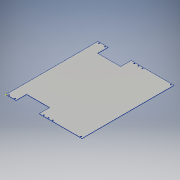
# Autodesk Inventor part: Belly Pan
Saved by Autodesk Inventor 2018 (Build 220112000, 112)
## iProperties
Created: 2018-01-27
Part Number: Belly Pan
Material: Aluminum 6061
Document SubType Name: Modeling
Designer: s-4000369
Density: 2.7 g/cm^3
Appearance: Aluminum - Flat
Mass: 1648.73 g
Surface Area: 4866.5 cm^2
Volume: 610.641 cm^3
Author: s-4000369
Autodesk Inventor part; units mm, degrees
ref_plane "YZ Plane" through (0, 0, 0) normal (1, 0, 0) x (0, 1, 0)
ref_plane "XZ Plane" through (0, 0, 0) normal (0, 1, 0) x (-1, 0, 0)
ref_plane "XY Plane" through (0, 0, 0) normal (0, 0, 1) x (1, 0, 0)
sketch "Sketch1" plane through (0, 0, 0) normal (0, 1, 0) x (-1, 0, 0)
  point P0 (0, 0)
sketch "Sketch2" plane through (0, 0, 0) normal (0, 1, 0) x (-1, 0, 0)
  line L0 (-61.9252, 0) -> (0, 0)
  line L1 (0, 0) -> (0, -558.8)
  line L2 (0, -558.8) -> (-61.9252, -558.8)
  line L3 (-61.9252, -558.8) -> (-61.9252, -495.3)
  line L4 (-61.9252, -495.3) -> (-201.6252, -495.3)
  line L5 (-201.6252, -495.3) -> (-201.6252, -558.8)
  line L6 (-201.6252, -558.8) -> (-461.9752, -558.8)
  line L7 (-461.9752, -558.8) -> (-461.9752, 0)
  line L8 (-461.9752, 0) -> (-201.6252, 0)
  line L9 (-201.6252, 0) -> (-201.6252, -63.5)
  line L10 (-201.6252, -63.5) -> (-61.9252, -63.5)
  line L11 (-61.9252, -63.5) -> (-61.9252, 0)
  point P0 (0, 0)
  dimension "d1" = 558.8
  dimension "d2" = 139.7
  dimension "d3" = 61.9252
  dimension "d4" = 63.5
  dimension "d8" = 260.35
  constraints: 24 end point, 8 perpendicular, 5 point on line, 2 collinear, 1 coincident, 1 horizontal, 1 vertical
  measures "d1" distance between parallel lines of L6 L8
  measures "d2" distance of L9.end L10.end
  measures "d3" distance of L0.start L0.end
  measures "d4" distance of L8.end L9.end
  measures "d8" distance of L7.end L8.end
extrude "Extrusion1" add sketch "Sketch2" along normal blind 1.5875
sketch "Sketch3" plane through (0, 1.5875, 0) normal (0, 1, 0) x (1, 0, 0)
  line L0 (461.9752, 0) -> (461.9752, 558.8) projected
  line L1 (461.9752, 0) -> (461.9752, 12.7)
  line L2 (461.9752, 12.7) -> (201.6252, 12.7)
  line L3 (201.6252, 63.5) -> (201.6252, 0) projected
  line L4 (201.6252, 558.8) -> (461.9752, 558.8) projected
  line L5 (461.9752, 558.8) -> (461.9752, 546.1)
  line L6 (461.9752, 546.1) -> (201.6252, 546.1)
  line L7 (201.6252, 558.8) -> (201.6252, 495.3) projected
  line L8 (461.9752, 6.35) -> (201.6252, 6.35)
  line L9 (461.9752, 552.45) -> (201.6252, 552.45)
  line L10 (461.9752, 552.45) -> (449.2752, 552.45)
  line L11 (461.9752, 6.35) -> (449.2752, 6.35)
  line L12 (201.6252, 552.45) -> (227.0252, 552.45)
  line L13 (227.0252, 552.45) -> (252.4252, 552.45)
  line L14 (252.4252, 552.45) -> (277.8252, 552.45)
  line L15 (201.6252, 6.35) -> (227.0252, 6.35)
  line L16 (227.0252, 6.35) -> (252.4252, 6.35)
  line L17 (252.4252, 6.35) -> (277.8252, 6.35)
  line L18 (0, 558.8) -> (0, 0) projected
  line L19 (0, 552.45) -> (62.0515, 552.45)
  line L20 (0, 6.35) -> (62.0515, 6.35)
  line L21 (0, 552.45) -> (12.7, 552.45)
  line L22 (61.9252, 495.3) -> (61.9252, 558.8) projected
  line L23 (61.9252, 552.45) -> (49.2252, 552.45)
  circle A0 centre (49.2252, 552.45) radius 3.2512
  circle A1 centre (12.7, 552.45) radius 3.2512
  circle A2 centre (227.0252, 552.45) radius 3.2512
  circle A3 centre (252.4252, 552.45) radius 3.2512
  circle A4 centre (277.8252, 552.45) radius 3.2512
  circle A5 centre (449.2752, 552.45) radius 3.2512
  line L24 (461.9752, 6.35) -> (449.2752, 6.35)
  circle A6 centre (449.2752, 6.35) radius 3.2512
  line L25 (201.6252, 6.35) -> (227.0252, 6.35)
  circle A7 centre (223.774, 6.35) radius 3.2512
  circle A8 centre (252.4252, 6.35) radius 3.2512
  circle A9 centre (277.8252, 6.35) radius 3.2512
  circle A10 centre (49.2252, 6.35) radius 3.2512
  circle A11 centre (12.7, 6.35) radius 3.2512
  line L26 (449.2752, 558.8) -> (449.2752, 0)
  line L27 (449.2752, 558.8) -> (455.6252, 558.8)
  line L28 (455.6252, 558.8) -> (455.6252, 0)
  line L29 (461.9752, 0) -> (201.6252, 0) projected
  line L30 (455.6252, 546.1) -> (455.6252, 368.3)
  line L31 (455.6252, 368.3) -> (455.6252, 190.5)
  circle A12 centre (455.6252, 368.3) radius 3.2512
  circle A13 centre (455.6252, 190.5) radius 3.2512
  dimension "d9" = 12.7
  dimension "d10" = 12.7
  dimension "d11" = 12.7
  dimension "d12" = 25.4
  dimension "d13" = 25.4
  dimension "d14" = 25.4
  dimension "d15" = 12.7
  dimension "d16" = 12.7
  dimension "d17" = 6.5024
  dimension "d18" = 12.7
  dimension "d19" = 177.8
  dimension "d20" = 177.8
  dimension "d21" = 6.5024
  constraints: 50 end point, 29 point on line, 14 centre point, 11 coincident, 5 perpendicular, 2 collinear, 2 horizontal, 2 midpoint, 1 vertical
  measures "d9" distance of L0.start L1.end
  measures "d10" distance of L0.end L5.end
  measures "d11" distance of L9.start L10.end
  measures "d12" distance of L9.end L12.end
  measures "d13" distance of L12.end L13.end
  measures "d14" distance of L13.end L14.end
  measures "d15" distance of L19.start L21.end
  measures "d16" distance of L23.start L23.end
  measures "d17" diameter of A0
  measures "d18" distance from line of L0 L11.end
  measures "d19" distance of L30.start L30.end
  measures "d20" distance of L30.end L31.end
  measures "d21" diameter of A12
extrude "Extrusion2" cut sketch "Sketch3" against normal blind 25.4 contours A6 L26 L8 | L8 L26 A6 | A6 L8 L26 | L8 A6 L26 | A9 L8 | L8 A9 | A7 L8 | L8 A7 | A5 L26 L9 | L9 L26 A5 | A5 L9 L26 | L9 A5 L26 | A8 L8 | L8 A8 | A2 L9 | L9 A2 | A4 L9 | L9 A4 | A3 L9 | L9 A3 | A10 L20 | L20 A10 | A11 L20 | L20 A11 | A0 L19 | L19 A0 | A1 L19 | L19 A1
body "Solid1"
